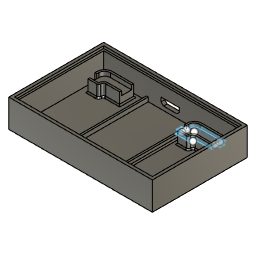
Keypad_1kGap_V3 (Autodesk Fusion 360 design; units mm, degrees)
Autodesk Fusion 360 part; units mm, degrees
sketch "Sketch1" plane through (0, 0, 0) normal (0, 0, 1) x (1, 0, 0) in component "Case"
  line L0 (-9.9826, 59.2) -> (4.0174, 59.2)
  line L1 (4.0174, 59.2) -> (4.0174, 45.2)
  line L2 (4.0174, 45.2) -> (-9.9826, 45.2)
  line L3 (-9.9826, 45.2) -> (-9.9826, 59.2)
  line L4 (4.0174, 45.2) -> (8.4507, 45.2) construction
  line L5 (22.4507, 45.2) -> (26.884, 45.2) construction
  line L6 (26.884, 45.2) -> (40.884, 45.2)
  line L7 (40.884, 45.2) -> (40.884, 59.2)
  line L8 (40.884, 59.2) -> (26.884, 59.2)
  line L9 (26.884, 59.2) -> (26.884, 45.2)
  line L10 (-11.284, 61.2) -> (42.1497, 61.2)
  line L11 (8.4507, 45.2) -> (22.4507, 45.2) construction
  line L12 (42.1497, 61.2) -> (15.4327, 61.2) construction
  line L13 (15.4327, 61.2) -> (24.5827, 61.2)
  line L14 (24.5827, 61.2) -> (24.5827, 27.8667)
  line L15 (24.5827, 27.8667) -> (15.4327, 27.8667)
  line L16 (24.5827, 27.8667) -> (6.2827, 27.8667)
  line L17 (6.2827, 27.8667) -> (6.2827, 61.2)
  line L18 (6.2827, 61.2) -> (24.5827, 61.2)
  line L19 (24.5827, 61.2) -> (24.5827, 27.8667)
  line L20 (25.3827, 61.2) -> (25.3827, 27.0667)
  line L21 (25.3827, 27.0667) -> (5.4827, 27.0667)
  line L22 (5.4827, 27.0667) -> (5.4827, 61.2)
  line L23 (-3.7837, 61.2) -> (-3.7837, 59.2) construction
  line L24 (34.3937, 59.2) -> (34.3937, 61.2) construction
  line L25 (40.884, 54.9257) -> (42.967, 54.9257) construction
  line L26 (-9.9826, 56.4827) -> (-12.0666, 56.4827) construction
  line L27 (42.967, 54.9257) -> (42.967, 61.2)
  line L28 (42.967, 61.2) -> (42.1497, 61.2)
  line L29 (-12.0666, 56.4827) -> (-12.0666, 61.2)
  line L30 (-12.0666, 61.2) -> (-11.284, 61.2)
  line L31 (-12.0666, 61.2) -> (42.967, 61.2)
  line L32 (42.967, 61.2) -> (42.967, 26.2)
  line L33 (42.967, 26.2) -> (-12.0666, 26.2)
  line L34 (-12.0666, 26.2) -> (-12.0666, 61.2)
  line L35 (-14.0666, 63.2) -> (44.967, 63.2)
  line L36 (44.967, 63.2) -> (44.967, 24.2)
  line L37 (44.967, 24.2) -> (-14.0666, 24.2)
  line L38 (-14.0666, 24.2) -> (-14.0666, 63.2)
  dimension "d1" = 14
  dimension "d2" = 14
  dimension "d3" = 4.4333
  dimension "d4" = 14
  dimension "d6" = 4.4333
  dimension "d7" = 14
  dimension "d8" = 14
  dimension "d19" = 26.717
  dimension "d21" = 9.15
  dimension "d22" = 33.3333
  dimension "d23" = 18.3
  dimension "d24" = 33.3333
  dimension "d25" = -0.8
  dimension "d60" = 2
  dimension "d61" = 2
  dimension "d62" = 2.083
  dimension "d63" = 2.084
  dimension "d64" = 35
  dimension "d65" = -2
  constraint horizontal L0
  constraint vertical L1
  constraint horizontal L2
  constraint vertical L3
  constraint perpendicular L1 L4
  constraint horizontal L6
  constraint vertical L7
  constraint horizontal L8
  constraint vertical L9
  constraint horizontal L10
  constraint parallel L5 L11
  constraint horizontal L13
  constraint vertical L14
  constraint horizontal L15
  constraint horizontal L16
  constraint vertical L17
  constraint horizontal L18
  constraint vertical L19
  constraint coincident L10 L23.start
  constraint coincident L0 L23.end
  constraint perpendicular L0 L23
  constraint coincident L8 L24.start
  constraint coincident L12 L24.end
  constraint coincident L10 L24.end
  constraint perpendicular L12 L24
  constraint coincident L7 L25.start
  constraint perpendicular L7 L25
  constraint coincident L3 L26.start
  constraint perpendicular L3 L26
  constraint perpendicular L10 L27
  constraint perpendicular L27 L28
  constraint perpendicular L10 L29
  constraint perpendicular L29 L30
  constraint horizontal L31
  constraint vertical L32
  constraint horizontal L33
  constraint vertical L34
  measures "d1" distance of L0.start L0.end
  measures "d2" distance of L0.start L2.end
  measures "d3" distance of L1.end L4.end
  measures "d4" distance of L4.end L5.start
  measures "d6" distance of L5.start L5.end
  measures "d7" distance of L5.end L6.end
  measures "d8" distance of L5.end L8.end
  measures "d19" distance of L10.end L12.end
  measures "d21" distance of L12.end L13.end
  measures "d22" distance of L13.end L14.end
  measures "d23" distance of L14.end L16.end
  measures "d24" distance of L14.end L13.end
  measures "d60" distance of L23.start L23.end
  measures "d61" distance of L24.start L24.end
  measures "d62" distance of L25.start L25.end
  measures "d63" distance of L26.start L26.end
  measures "d64" distance of L29.end L33.end
extrude "Extrude1" add sketch "Sketch1" against normal blind 2 contours L0 L1 L2 L3 | L6 L7 L8 L9 | L10 L20 L21 L22 L27 L28 L29 L30 L31 L32 L33 L34 | L10 L14 L15 L16 L17 L19 L20 L21 L22 L31 | L10 L13 L14 L15 L16 L17 L18 L19 L31 | L35 L36 L37 L38 makes body 1 in component "Case"
extrude "Extrude2" add sketch "Sketch1" along normal blind 1.7 contours L10 L14 L15 L16 L17 L19 L20 L21 L22 L31 bodies 1 in component "Case"
extrude "Extrude3" add sketch "Sketch1" along normal blind 10 contours L35 L36 L37 L38 bodies 1 in component "Case"
chamfer "Chamfer1" distance 0.5 angle 45 3 edges at (25.3827, 44.1333, 0) (5.4827, 44.1333, 0) (15.4327, 27.0667, 0) on bodies 1 in component "Case"
ref_plane "WorkPlane1" through (15.4327, 44.1333, 1.7) normal (0, 0, 1) x (1, 0, 0) in component "Case"
sketch "Sketch2" plane through (15.4328, 43.7, 1.7) normal (0, 0, 1) x (1, 0, 0) in component "Case"
  line L0 (-27.4995, 17.5) -> (27.5342, 17.5)
  line L1 (-9.1502, 17.5) -> (-9.1502, -15.8333)
  line L2 (-9.1502, -15.8333) -> (9.1498, -15.8333)
  line L3 (9.1498, -15.8333) -> (9.1498, 17.5)
  line L4 (27.5342, -17.5) -> (-27.4995, -17.5)
  line L5 (-27.4995, -17.5) -> (-27.4995, 17.5)
  line L6 (27.5342, 17.5) -> (27.5342, -17.5)
  line L7 (-29.4995, -19.5) -> (29.5342, -19.5)
  line L8 (29.5342, -19.5) -> (29.5342, 19.5)
  line L9 (29.5342, 19.5) -> (-29.4995, 19.5)
  line L10 (-29.4995, 19.5) -> (-29.4995, -19.5)
  line L11 (9.1498, 17.5) -> (-9.1502, 17.5)
  line L12 (-9.1502, 17.5) -> (-3.9002, 17.5) construction
  line L13 (-3.9002, 17.5) -> (3.5998, 17.5)
  line L14 (3.5998, 17.5) -> (3.5998, 20.5)
  line L15 (3.5998, 20.5) -> (-3.9002, 20.5)
  line L16 (-3.9002, 20.5) -> (-3.9002, 17.5)
  dimension "d66" = 5.25
  dimension "d67" = 7.5
  dimension "d68" = 3
  constraint coincident L1.start L11.end
  constraint perpendicular L1 L12
  constraint horizontal L13
  constraint vertical L14
  constraint horizontal L15
  constraint vertical L16
  measures "d66" distance of L1.start L12.end
  measures "d67" distance of L12.end L13.end
  measures "d68" distance of L12.end L15.end
extrude "Extrude4" cut sketch "Sketch2" along normal blind 2.6 and the other way blind 0.1 contours L0 L9 L11 L13 L14 L16 | L9 L14 L15 L16 bodies 1 in component "Case"
chamfer "Chamfer2" distance 1 angle 45 2 edges at (11.5327, 62.2, 1.6) (19.0327, 62.2, 1.6) on bodies 1 in component "Case"
sketch "Sketch1 (2)" plane through (0, 63.2, 0) normal (0, 1, 0) x (-1, 0, 0)
  line L0 (-12.5327, 1.6) -> (-18.0327, 1.6)
  line L1 (-18.0327, 1.6) -> (-19.0327, 2.6)
  line L2 (-19.0327, 2.6) -> (-19.0327, 4.3)
  line L3 (-19.0327, 4.3) -> (-11.5327, 4.3)
  line L4 (-11.5327, 4.3) -> (-11.5327, 2.6)
  line L5 (-11.5327, 2.6) -> (-12.5327, 1.6)
  line L6 (-44.967, 10) -> (-44.967, -2)
  line L7 (-44.967, -2) -> (14.0666, -2)
  line L8 (14.0666, -2) -> (14.0666, 10)
  line L9 (14.0666, 10) -> (-44.967, 10)
  line L10 (-10.5327, 2.1858) -> (-12.1185, 0.6)
  line L11 (-12.1185, 0.6) -> (-18.4469, 0.6)
  line L12 (-18.4469, 0.6) -> (-20.0327, 2.1858)
  line L13 (-20.0327, 2.1858) -> (-20.0327, 5.3)
  line L14 (-20.0327, 5.3) -> (-10.5327, 5.3)
  line L15 (-10.5327, 5.3) -> (-10.5327, 2.1858)
  dimension "d69" = -1
  measures "d69" distance of L5
extrude "Extrude5" cut sketch "Sketch1 (2)" against normal blind 0.5 contours L10 L11 L12 L13 L14 L15 bodies 1 in component "Case"
fillet "Fillet1" radius 0.5 12 edges at (19.2398, 62.7, 1.3929) (19.2398, 63.2, 1.3929) (20.0327, 62.7, 3.7429) (20.0327, 63.2, 3.7429) (15.2827, 62.7, 0.6) (15.2827, 63.2, 0.6) (11.3256, 62.7, 1.3929) (11.3256, 63.2, 1.3929) (10.5327, 62.7, 3.7429) (10.5327, 63.2, 3.7429) (15.2827, 62.7, 5.3) (15.2827, 63.2, 5.3) on bodies 1 in component "Case"
sketch "Sketch2 (2)" plane through (0, 0, 10) normal (0, 0, 1) x (-1, 0, 0)
  line L0 (-42.967, -26.2) -> (12.0666, -26.2)
  line L1 (12.0666, -26.2) -> (12.0666, -61.2)
  line L2 (12.0666, -61.2) -> (-42.967, -61.2)
  line L3 (-42.967, -61.2) -> (-42.967, -26.2)
  line L4 (14.0666, -24.2) -> (-44.967, -24.2)
  line L5 (-44.967, -24.2) -> (-44.967, -63.2)
  line L6 (-44.967, -63.2) -> (14.0666, -63.2)
  line L7 (14.0666, -63.2) -> (14.0666, -24.2)
  line L8 (12.8666, -25.4) -> (12.8666, -62)
  line L9 (12.8666, -62) -> (-43.767, -62)
  line L10 (-43.767, -62) -> (-43.767, -25.4)
  line L11 (-43.767, -25.4) -> (12.8666, -25.4)
  dimension "d72" = -0.8
extrude "Extrude6" cut sketch "Sketch2 (2)" against normal blind 1 contours L8 L9 L10 L11 bodies 1 in component "Case"
sketch "Sketch3" plane through (0, 0, 10) normal (0, 0, 1) x (-1, 0, 0)
  line L0 (12.8666, -62) -> (-43.767, -62)
  line L1 (-43.767, -62) -> (-43.767, -25.4)
  line L2 (-43.767, -25.4) -> (12.8666, -25.4)
  line L3 (12.8666, -25.4) -> (12.8666, -62)
  line L4 (14.0666, -24.2) -> (-44.967, -24.2)
  line L5 (-44.967, -24.2) -> (-44.967, -63.2)
  line L6 (-44.967, -63.2) -> (14.0666, -63.2)
  line L7 (14.0666, -63.2) -> (14.0666, -24.2)
  line L8 (12.7666, -25.5) -> (12.7666, -61.9)
  line L9 (12.7666, -61.9) -> (-43.667, -61.9)
  line L10 (-43.667, -61.9) -> (-43.667, -25.5)
  line L11 (-43.667, -25.5) -> (12.7666, -25.5)
  line L12 (12.0666, -61.2) -> (-42.967, -61.2)
  line L13 (-42.967, -61.2) -> (-42.967, -26.2)
  line L14 (-42.967, -26.2) -> (12.0666, -26.2)
  line L15 (12.0666, -26.2) -> (12.0666, -61.2)
  line L16 (-43.767, -25.4) -> (-43.767, -62)
  line L17 (-43.767, -62) -> (12.8666, -62)
  line L18 (12.8666, -62) -> (12.8666, -25.4)
  line L19 (12.8666, -25.4) -> (-43.767, -25.4)
  dimension "d73" = 0.1
extrude "Extrude1'" add sketch "Sketch3" against normal blind 0.8 separate body contours L8 L9 L10 L11 makes body 2 in component "lid"
sketch "Sketch4" plane through (0, 0, 10) normal (0, 0, 1) x (-1, 0, 0)
  line L0 (12.8666, -62) -> (-43.767, -62)
  line L1 (-43.767, -62) -> (-43.767, -25.4)
  line L2 (-43.767, -25.4) -> (12.8666, -25.4)
  line L3 (12.8666, -25.4) -> (12.8666, -62)
  line L4 (14.0666, -24.2) -> (-44.967, -24.2)
  line L5 (-44.967, -24.2) -> (-44.967, -63.2)
  line L6 (-44.967, -63.2) -> (14.0666, -63.2)
  line L7 (14.0666, -63.2) -> (14.0666, -24.2)
  line L8 (-44.967, -63.2) -> (14.0666, -63.2)
  line L9 (14.0666, -63.2) -> (14.0666, -24.2)
  line L10 (14.0666, -24.2) -> (-44.967, -24.2)
  line L11 (-44.967, -24.2) -> (-44.967, -63.2)
  constraint horizontal L8
  constraint vertical L9
  constraint horizontal L10
  constraint vertical L11
  constraint coincident L4.start L7.end
  constraint coincident L5.end L6.start
extrude "Extrude2'" add sketch "Sketch4" along normal blind 1.5 contours L0 L1 L2 L3 | L4 L5 L6 L7 L8 L9 L10 L11 bodies 2 in component "lid"
extrude "Extrude3'" cut sketch "Sketch1" along normal blind 23 contours L0 L1 L2 L3 | L6 L7 L8 L9 bodies 2 in component "lid"
chamfer "Chamfer1'" distance 0.25 angle 45 8 edges at (33.884, 59.2, 11.5) (40.884, 52.2, 11.5) (33.884, 45.2, 11.5) (26.884, 52.2, 11.5) (4.0174, 52.2, 11.5) (-2.9826, 59.2, 11.5) (-9.9826, 52.2, 11.5) (-2.9826, 45.2, 11.5) on bodies 2 in component "lid"
chamfer "Chamfer2'" distance 0.5 angle 45 4 edges at (15.4502, 24.2, 11.5) (44.967, 43.7, 11.5) (15.4502, 63.2, 11.5) (-14.0666, 43.7, 11.5) on bodies 2 in component "lid"
chamfer "Chamfer3" distance 0.5 angle 45 4 edges at (15.4502, 24.2, -2) (44.967, 43.7, -2) (15.4502, 63.2, -2) (-14.0666, 43.7, -2) on bodies 1 in component "Case"
ref_plane "WorkPlane2" through (15.4502, 43.7, 3.4) normal (0, 0, 1) x (1, 0, 0) in component "Case"
sketch "Sketch5" plane through (15.4502, 43.7, 3.4) normal (0, 0, 1) x (1, 0, 0) in component "Case"
  line L0 (-27.5168, 17.5) -> (27.5168, 17.5)
  line L1 (27.5168, 17.5) -> (27.5168, -17.5)
  line L2 (27.5168, -17.5) -> (-27.5168, -17.5)
  line L3 (-27.5168, -17.5) -> (-27.5168, 17.5)
  line L4 (28.3168, -18.3) -> (28.3168, 18.3)
  line L5 (28.3168, 18.3) -> (-28.3168, 18.3)
  line L6 (-28.3168, 18.3) -> (-28.3168, -18.3)
  line L7 (-28.3168, -18.3) -> (28.3168, -18.3)
  line L8 (-28.3168, 18.3) -> (28.3168, 18.3)
  line L9 (28.3168, 18.3) -> (28.3168, -18.3)
  line L10 (28.3168, -18.3) -> (-28.3168, -18.3)
  line L11 (-28.3168, -18.3) -> (-28.3168, 18.3)
  line L12 (-29.5168, -19.5) -> (29.5168, -19.5)
  line L13 (29.5168, -19.5) -> (29.5168, 19.5)
  line L14 (29.5168, 19.5) -> (-29.5168, 19.5)
  line L15 (-29.5168, 19.5) -> (-29.5168, -19.5)
  line L16 (-20.1287, 17.5) -> (-20.1287, 15.083) construction
  line L17 (-15.1433, 17.5) -> (-15.1433, 15.083) construction
  line L18 (-27.5013, 11.953) -> (-24.7083, 11.953) construction
  line L19 (-27.5013, 11.953) -> (-27.5168, 17.5) construction
  line L20 (-27.5013, 11.953) -> (-27.5013, 9.253) construction
  line L21 (-27.5013, 9.253) -> (-24.7083, 9.253) construction
  line L22 (-24.7083, 9.253) -> (-21.3083, 9.253)
  line L23 (-24.7083, 9.253) -> (-24.7083, 12.853)
  line L24 (-21.3083, 9.253) -> (-19.4083, 9.253) construction
  line L25 (-19.4083, 9.253) -> (-19.4083, 11.153) construction
  line L26 (-19.4083, 11.153) -> (-13.7883, 11.153)
  line L27 (-13.7883, 11.153) -> (-13.7883, 15.083)
  line L28 (-13.7883, 15.083) -> (-22.3883, 15.083)
  arc A0 (-22.3883, 15.083) -> (-24.7083, 12.853) centre (-22.4765, 12.853) ccw
  arc A1 (-19.4083, 11.153) -> (-21.3083, 9.253) centre (-19.4083, 9.253) ccw
  arc A2 (-22.3863, 15.183) -> (-24.8083, 12.853) centre (-22.4765, 12.853) ccw
  line L29 (-24.8083, 9.153) -> (-24.8083, 12.853)
  line L30 (-24.8083, 9.153) -> (-21.2055, 9.153)
  arc A3 (-19.4083, 11.053) -> (-21.2055, 9.153) centre (-19.4083, 9.253) ccw
  line L31 (-19.4083, 11.053) -> (-13.6883, 11.053)
  line L32 (-13.6883, 11.053) -> (-13.6883, 15.183)
  line L33 (-13.6883, 15.183) -> (-22.3863, 15.183)
  line L34 (-25.6083, 8.353) -> (-19.8442, 8.353)
  arc A4 (-19.4083, 10.253) -> (-19.8442, 8.353) centre (-19.4083, 9.253) ccw
  line L35 (-19.4083, 10.253) -> (-12.8883, 10.253)
  line L36 (-12.8883, 10.253) -> (-12.8883, 15.983)
  line L37 (-12.8883, 15.983) -> (-22.372, 15.983)
  arc A5 (-22.372, 15.983) -> (-25.6083, 12.853) centre (-22.4765, 12.853) ccw
  line L38 (-25.6083, 8.353) -> (-25.6083, 12.853)
  line L39 (-13.6883, 11.053) -> (-13.6883, 12.683) construction
  line L40 (-13.6883, 12.683) -> (-11.6883, 12.683)
  line L41 (-11.6883, 12.683) -> (-11.6883, 14.483)
  line L42 (-11.6883, 14.483) -> (-13.6883, 14.483)
  line L43 (-13.6883, 14.483) -> (-13.6883, 12.683)
  line L44 (-24.8083, 9.153) -> (-24.8083, 10.153) construction
  line L45 (-24.8083, 10.153) -> (-26.8083, 10.153)
  line L46 (-26.8083, 10.153) -> (-26.8083, 11.953)
  line L47 (-26.8083, 11.953) -> (-24.8083, 11.953)
  line L48 (-24.8083, 11.953) -> (-24.8083, 10.153)
  line L49 (-13.6883, 11.053) -> (-13.6883, 10.253)
  line L50 (-13.6883, 15.183) -> (-13.6883, 15.983)
  line L51 (-24.8083, 9.153) -> (-24.8083, 8.353)
  dimension "d77" = 2.417
  dimension "d78" = 2.417
  dimension "d79" = 2.793
  dimension "d81" = 5.547
  dimension "d82" = 2.7
  dimension "d83" = 2.793
  dimension "d84" = 3.4
  dimension "d85" = 3.6
  dimension "d86" = 1.9
  dimension "d87" = 1.9
  dimension "d88" = 5.62
  dimension "d89" = 3.93
  dimension "d90" = 8.6
  dimension "d91" = 0.1
  dimension "d92" = -0.9
  dimension "d93" = 1.63
  dimension "d94" = 2
  dimension "d95" = 1.8
  dimension "d96" = 1
  dimension "d97" = 2
  dimension "d98" = 1.8
  constraint coincident L0 L16.start
  constraint perpendicular L0 L16
  constraint coincident L0 L17.start
  constraint perpendicular L0 L17
  constraint perpendicular L3 L18
  constraint coincident L0.start L3.end
  constraint perpendicular L18 L20
  constraint perpendicular L20 L21
  constraint parallel L21 L22
  constraint perpendicular L22 L23
  constraint parallel L22 L24
  constraint perpendicular L24 L25
  constraint perpendicular L25 L26
  constraint perpendicular L26 L27
  constraint perpendicular L27 L28
  constraint tangent L23 A0
  constraint tangent L26 A1
  constraint perpendicular L31 L39
  constraint horizontal L40
  constraint vertical L41
  constraint horizontal L42
  constraint vertical L43
  constraint perpendicular L21 L44
  constraint horizontal L45
  constraint vertical L46
  constraint horizontal L47
  constraint vertical L48
  constraint coincident L35 L49.end
  constraint perpendicular L35 L49
  constraint coincident L37 L50.end
  constraint perpendicular L37 L50
  constraint coincident L34 L51.end
  constraint perpendicular L34 L51
  measures "d77" distance of L16.start L16.end
  measures "d78" distance of L17.start L17.end
  measures "d79" distance of L18.start L18.end
  measures "d81" vertical distance of L18.start L0.start
  measures "d82" distance of L18.start L20.end
  measures "d83" distance of L20.end L21.end
  measures "d84" distance of L21.end L22.end
  measures "d85" distance of L21.end L23.end
  measures "d86" distance of L22.end L24.end
  measures "d87" distance of L24.end L25.end
  measures "d88" distance of L25.end L26.end
  measures "d89" distance of L26.end L27.end
  measures "d90" distance of L27.end L28.end
  measures "d93" distance of L31.end L39.end
  measures "d94" distance of L39.end L40.end
  measures "d95" distance of L39.end L42.end
  measures "d96" distance of L29.start L44.end
  measures "d97" distance of L44.end L45.end
  measures "d98" distance of L44.end L47.end
extrude "Extrude7" add sketch "Sketch5" along normal blind -3.4 and the other way blind -1.5 contours A2 L29 L33 L37 A5 L38 L47 L50 | L30 A3 L31 L34 A4 L35 L49 L51 bodies 1 in component "Case"
extrude "Extrude8" add sketch "Sketch5" along normal blind -3.4 and the other way blind 0.25 contours L22 L23 L26 L27 L28 A0 A1 | A2 L29 L30 A3 L31 L32 L33 L43 L48 bodies 1 in component "Case"
fillet "Fillet2" radius 0.8 1 edges at (-4.394, 52.053, 2.45) on bodies 1 in component "Case"
sketch "Sketch6" plane through (15.4502, 43.7, 3.4) normal (0, 0, 1) x (1, 0, 0) in component "Case"
  line L0 (17.4577, 10.253) -> (23.9777, 10.253)
  line L1 (17.4577, 11.053) -> (23.1777, 11.053)
  arc A0 (17.4577, 11.053) -> (15.6605, 9.153) centre (17.4577, 9.253) ccw
  arc A1 (17.4577, 10.253) -> (17.0218, 8.353) centre (17.4577, 9.253) ccw
  line L2 (11.2577, 8.353) -> (17.0218, 8.353)
  line L3 (12.0577, 9.153) -> (15.6605, 9.153)
  line L4 (11.2577, 8.353) -> (11.2577, 12.853)
  line L5 (12.0577, 9.153) -> (12.0577, 12.853)
  line L6 (12.0577, 10.153) -> (10.0577, 10.153)
  line L7 (10.0577, 11.953) -> (12.0577, 11.953)
  line L8 (10.0577, 10.153) -> (10.0577, 11.953)
  arc A2 (14.4797, 15.183) -> (12.0577, 12.853) centre (14.3895, 12.853) ccw
  arc A3 (14.494, 15.983) -> (11.2577, 12.853) centre (14.3895, 12.853) ccw
  line L9 (23.9777, 15.983) -> (14.494, 15.983)
  line L10 (23.1777, 15.183) -> (14.4797, 15.183)
  line L11 (23.9777, 10.253) -> (23.9777, 15.983)
  line L12 (23.1777, 11.053) -> (23.1777, 15.183)
  line L13 (23.1777, 15.183) -> (23.1777, 15.983)
  line L14 (23.1777, 11.053) -> (23.1777, 10.253)
  line L15 (12.0577, 9.153) -> (12.0577, 8.353)
  line L16 (25.1777, 12.683) -> (25.1777, 14.483)
  line L17 (23.1777, 12.683) -> (25.1777, 12.683)
  line L18 (25.1777, 14.483) -> (23.1777, 14.483)
  dimension "d109" = 1.63
  dimension "d110" = 2
  dimension "d111" = 1.8
  dimension "d112" = 1
  dimension "d113" = 2
  dimension "d114" = 1.8
  constraint horizontal L17
  constraint vertical L16
  constraint horizontal L18
  constraint horizontal L6
  constraint vertical L8
  constraint horizontal L7
  constraint coincident L14.end L0
  constraint perpendicular L0 L14
  constraint coincident L13.end L9
  constraint perpendicular L9 L13
  constraint coincident L15.end L2
  constraint perpendicular L2 L15
  measures "d109" distance of L1.end L17.start
  measures "d110" distance of L16.start L17.start
  measures "d111" distance of L17.start L18.end
  measures "d112" distance of L3.start L6.start
  measures "d113" distance of L6.end L6.start
  measures "d114" distance of L7.end L6.start
extrude "Extrude9" add sketch "Sketch6" along normal blind -3.4 and the other way blind -1.5 contours L0 L1 A0 A1 L2 L3 L14 L15 | L4 L5 L7 A2 A3 L9 L10 L13 bodies 1 in component "Case"
extrude "Extrude10" add sketch "Sketch6" along normal blind -3.4 and the other way blind 0.25 contours L1 A0 L3 L5 A2 L10 L12 bodies 1 in component "Case"
fillet "Fillet3" radius 0.8 1 edges at (32.472, 52.053, 2.45) on bodies 1 in component "Case"
chamfer "Chamfer4" distance 0.5 angle 45 20 edges at (29.3093, 52.053, 0) (31.6919, 52.3033, 0) (32.1814, 53.6402, 0) (35.7679, 53.953, 0) (38.6279, 56.818, 0) (27.5079, 53.853, 0) (27.1079, 55.653, 0) (26.7079, 56.103, 0) (27.6625, 58.8041, 0) (34.2861, 59.683, 0) (-1.0981, 53.953, 0) (-4.6846, 53.6402, 0) (-5.1741, 52.3033, 0) (-7.5567, 52.053, 0) (1.7619, 56.818, 0) (-9.3581, 53.853, 0) (-9.2035, 58.8041, 0) (-10.1581, 56.103, 0) (-9.7581, 55.653, 0) (-2.5799, 59.683, 0) on bodies 1 in component "Case"
component "Case" placed x (1, 0, 0) y (0, 1, 0) z (0, 0, 1) at (0, 0, 0)
component "lid" placed x (1, 0, 0) y (0, 1, 0) z (0, 0, 1) at (0, 0, 0)
equation "d19 = 53.434 mm / 2"
equation "d21 = ( 18.3 / 2 ) * 1 mm"
equation "d74 = 10 mm - 6.6 mm"
